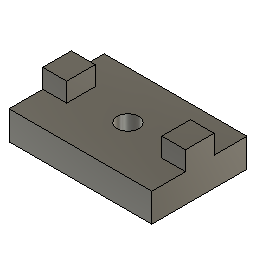
endstop linear rails v1 (Autodesk Fusion 360 design; units mm, degrees)
Autodesk Fusion 360 part; units mm, degrees
sketch "Skizze1" plane through (0, 0, 0) normal (0, 0, 1) x (1, 0, 0)
  line L0 (0, 0) -> (30, 0)
  line L1 (30, 0) -> (30, 20)
  line L2 (30, 20) -> (0, 20)
  line L3 (0, 20) -> (0, 0)
  dimension "d1" = 30
  dimension "d2" = 20
  constraint horizontal L0
  constraint vertical L1
  constraint horizontal L2
  constraint vertical L3
  constraint coincident L0.start L3.end
  measures "d1" distance of L0.start L0.end
  measures "d2" distance of L0.start L2.end
extrude "Extrusion1" add sketch "Skizze1" along normal blind 6
sketch "Skizze2" plane through (0, 0, 6) normal (0, 0, 1) x (-1, 0, 0)
  line L0 (0, -20) -> (0, 0)
  line L1 (0, 0) -> (-30, 0)
  line L2 (-30, 0) -> (-30, -20)
  line L3 (-30, -20) -> (0, -20)
  line L4 (0, -13.0831) -> (-30, -13.0831)
  line L5 (-30, -13.0831) -> (-30, -7.0831)
  line L6 (-30, -7.0831) -> (0, -7.0831)
  line L7 (0, -7.0831) -> (0, -13.0831)
  dimension "d5" = 30
  dimension "d6" = 6
  constraint horizontal L4
  constraint vertical L5
  constraint horizontal L6
  constraint vertical L7
  constraint coincident L0 L4.start
  measures "d5" distance of L4.start L4.end
  measures "d6" distance of L4.start L6.end
extrude "Extrusion2" add sketch "Skizze2" along normal blind 4 contours L0 L2 L4 L5 L6 L7
sketch "Skizze3" plane through (0, 0, 10) normal (0, 0, 1) x (-1, 0, 0)
  line L0 (0, -7.0831) -> (-30, -7.0831)
  line L1 (-30, -7.0831) -> (-30, -13.0831)
  line L2 (-30, -13.0831) -> (0, -13.0831)
  line L3 (0, -13.0831) -> (0, -7.0831)
  line L4 (-5.028, -13.0831) -> (-25.028, -13.0831)
  line L5 (-25.028, -13.0831) -> (-25.028, -7.0831)
  line L6 (-25.028, -7.0831) -> (-5.028, -7.0831)
  line L7 (-5.028, -7.0831) -> (-5.028, -13.0831)
  dimension "d9" = 20
  dimension "d10" = 6
  constraint horizontal L4
  constraint vertical L5
  constraint horizontal L6
  constraint vertical L7
  constraint coincident L2 L4.end
  measures "d9" distance of L4.start L4.end
  measures "d10" distance of L4.start L6.end
extrude "Extrusion3" cut sketch "Skizze3" against normal blind 4 contours L0 L2 L4 L5 L6 L7
sketch "Skizze4" plane through (0, 0, 6) normal (0, 0, 1) x (-1, 0, 0)
  line L0 (0, -13.0831) -> (-5.028, -13.0831)
  line L1 (-5.028, -13.0831) -> (-5.028, -7.0831)
  line L2 (-5.028, -7.0831) -> (0, -7.0831)
  line L3 (0, -7.0831) -> (0, 0)
  line L4 (0, 0) -> (-30, 0)
  line L5 (-30, 0) -> (-30, -7.0831)
  line L6 (-30, -7.0831) -> (-25.028, -7.0831)
  line L7 (-25.028, -7.0831) -> (-25.028, -13.0831)
  line L8 (-25.028, -13.0831) -> (-30, -13.0831)
  line L9 (-30, -13.0831) -> (-30, -20)
  line L10 (-30, -20) -> (0, -20)
  line L11 (0, -20) -> (0, -13.0831)
  circle A0 centre (-15, -10) radius 2.25
  dimension "d13" = 4.5
  measures "d13" diameter of A0
extrude "Extrusion4" cut sketch "Skizze4" against normal blind 6 contours A0
